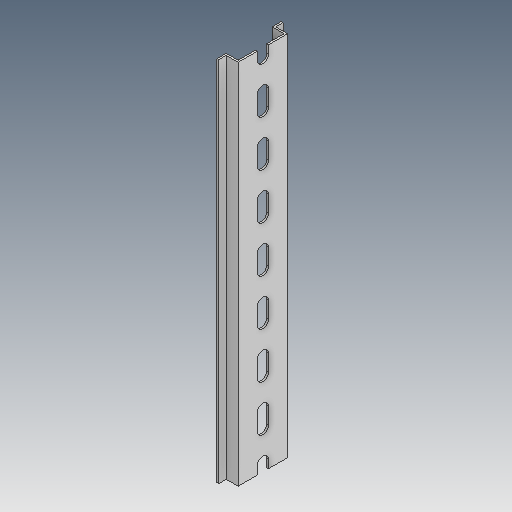
# Autodesk Inventor part: din_rail
Saved by Autodesk Inventor 2025.4 (Build 294407020, 407B)
## iProperties
Created: 2026-09-16
Part Number: din_rail
Material: Generic
Document SubType Name: Modeling
Designer: Aiden
Density: 1 g/cm^3
Appearance: Default
Author: Aiden
Autodesk Inventor part; units mm, degrees
ref_plane "YZ Plane" through (0, 0, 0) normal (1, 0, 0) x (0, 1, 0)
ref_plane "XZ Plane" through (0, 0, 0) normal (0, 1, 0) x (-1, 0, 0)
ref_plane "XY Plane" through (0, 0, 0) normal (0, 0, 1) x (1, 0, 0)
sketch "Sketch1" plane through (0, 0, 0) normal (0, 1, 0) x (-1, 0, 0)
  line L0 (0, 0) -> (0, -13.5)
  line L1 (0, -13.5) -> (6.5, -13.5)
  line L2 (6.5, -13.5) -> (6.5, -17.5)
  line L3 (1, 0) -> (1, -12.5)
  line L4 (1, -12.5) -> (7.5, -12.5)
  line L5 (7.5, -12.5) -> (7.5, -17.5)
  line L6 (7.5, -17.5) -> (6.5, -17.5)
  line L7 (1, 0) -> (0, 0) construction
  line L8 (0, 0) -> (0, 13.5)
  line L9 (0, 13.5) -> (6.5, 13.5)
  line L10 (6.5, 13.5) -> (6.5, 17.5)
  line L11 (1, 0) -> (1, 12.5)
  line L12 (1, 12.5) -> (7.5, 12.5)
  line L13 (7.5, 12.5) -> (7.5, 17.5)
  line L14 (7.5, 17.5) -> (6.5, 17.5)
  dimension "d0" = 13.5
  dimension "d1" = 1
  dimension "d2" = 7.5
  dimension "d3" = 17.5
  constraints: 30 end point, 6 symmetric about line, 3 horizontal, 2 vertical, 2 other
  measures "d0" distance of L0.start L0.end
  measures "d1" distance between parallel lines of L0 L3
  measures "d2" distance between parallel lines of L0 L5
  measures "d3" vertical distance of L2.end L0.start
extrude "Extrusion1" add sketch "Sketch1" along normal blind 200
sketch "Sketch2" plane through (-1, 0, -12.5) normal (-1, 0, 0) x (0, 0, 1)
  line L0 (0, 0) -> (25, 0) projected
  line L1 (25, 0) -> (25, 200) projected
  line L2 (0, 200) -> (25, 200) projected
  line L3 (0, 0) -> (0, 200) projected
  line L4 (25, 0) -> (25, 200) projected
  line L5 (12.5, 104.4) -> (12.5, 95.6) construction
  line L6 (30, 0) -> (30, 200) projected
  line L7 (9.4, 104.4) -> (9.4, 95.6)
  line L8 (15.6, 95.6) -> (15.6, 104.4)
  arc A0 (15.6, 104.4) -> (9.4, 104.4) centre (12.5, 104.4) ccw
  arc A1 (9.4, 95.6) -> (15.6, 95.6) centre (12.5, 95.6) ccw
  line L9 (12.5, 129.4) -> (12.5, 120.6) construction
  line L10 (9.4, 129.4) -> (9.4, 120.6)
  line L11 (15.6, 120.6) -> (15.6, 129.4)
  arc A2 (15.6, 129.4) -> (9.4, 129.4) centre (12.5, 129.4) ccw
  arc A3 (9.4, 120.6) -> (15.6, 120.6) centre (12.5, 120.6) ccw
  line L12 (12.5, 79.4) -> (12.5, 70.6) construction
  line L13 (9.4, 79.4) -> (9.4, 70.6)
  line L14 (15.6, 70.6) -> (15.6, 79.4)
  arc A4 (15.6, 79.4) -> (9.4, 79.4) centre (12.5, 79.4) ccw
  arc A5 (9.4, 70.6) -> (15.6, 70.6) centre (12.5, 70.6) ccw
  line L15 (12.5, 154.4) -> (12.5, 145.6) construction
  line L16 (9.4, 154.4) -> (9.4, 145.6)
  line L17 (15.6, 145.6) -> (15.6, 154.4)
  arc A6 (15.6, 154.4) -> (9.4, 154.4) centre (12.5, 154.4) ccw
  arc A7 (9.4, 145.6) -> (15.6, 145.6) centre (12.5, 145.6) ccw
  line L18 (12.5, 54.4) -> (12.5, 45.6) construction
  line L19 (9.4, 54.4) -> (9.4, 45.6)
  line L20 (15.6, 45.6) -> (15.6, 54.4)
  arc A8 (15.6, 54.4) -> (9.4, 54.4) centre (12.5, 54.4) ccw
  arc A9 (9.4, 45.6) -> (15.6, 45.6) centre (12.5, 45.6) ccw
  line L21 (12.5, 179.4) -> (12.5, 170.6) construction
  line L22 (9.4, 179.4) -> (9.4, 170.6)
  line L23 (15.6, 170.6) -> (15.6, 179.4)
  arc A10 (15.6, 179.4) -> (9.4, 179.4) centre (12.5, 179.4) ccw
  arc A11 (9.4, 170.6) -> (15.6, 170.6) centre (12.5, 170.6) ccw
  line L24 (12.5, 29.4) -> (12.5, 20.6) construction
  line L25 (9.4, 29.4) -> (9.4, 20.6)
  line L26 (15.6, 20.6) -> (15.6, 29.4)
  arc A12 (15.6, 29.4) -> (9.4, 29.4) centre (12.5, 29.4) ccw
  arc A13 (9.4, 20.6) -> (15.6, 20.6) centre (12.5, 20.6) ccw
  line L27 (12.5, 204.4) -> (12.5, 195.6) construction
  line L28 (9.4, 204.4) -> (9.4, 195.6)
  line L29 (15.6, 195.6) -> (15.6, 204.4)
  arc A14 (15.6, 204.4) -> (9.4, 204.4) centre (12.5, 204.4) ccw
  arc A15 (9.4, 195.6) -> (15.6, 195.6) centre (12.5, 195.6) ccw
  line L30 (12.5, 4.4) -> (12.5, -4.4) construction
  line L31 (9.4, 4.4) -> (9.4, -4.4)
  line L32 (15.6, -4.4) -> (15.6, 4.4)
  arc A16 (15.6, 4.4) -> (9.4, 4.4) centre (12.5, 4.4) ccw
  arc A17 (9.4, -4.4) -> (15.6, -4.4) centre (12.5, -4.4) ccw
  point P0 (12.5, 0)
  point P1 (12.5, 100)
  point P2 (12.5, 200)
  point P3 (25, 100)
  point P4 (12.5, 107.5)
  point P5 (12.5, 92.5)
  point P6 (12.5, 132.5)
  point P7 (12.5, 117.5)
  point P8 (12.5, 125)
  point P9 (12.5, 82.5)
  point P10 (12.5, 67.5)
  point P11 (12.5, 75)
  point P12 (12.5, 157.5)
  point P13 (12.5, 142.5)
  point P14 (12.5, 150)
  point P15 (12.5, 57.5)
  point P16 (12.5, 42.5)
  point P17 (12.5, 50)
  point P18 (12.5, 182.5)
  point P19 (12.5, 167.5)
  point P20 (12.5, 175)
  point P21 (12.5, 32.5)
  point P22 (12.5, 17.5)
  point P23 (12.5, 25)
  point P24 (12.5, 207.5)
  point P25 (12.5, 192.5)
  point P26 (12.5, 200)
  point P27 (12.5, 7.5)
  point P28 (12.5, -7.5)
  point P29 (12.5, 0)
  point P30 (9.4, 0)
  point P31 (15.6, 0)
  dimension "d6" = 6.2
  dimension "d7" = 15
  dimension "d10" = 25
  constraints: 72 end point, 38 point on circle, 18 centre point, 4 tangent, 3 midpoint, 2 parallel, 1 horizontal alignment, 1 vertical, 1 vertical alignment, 112 other
  measures "d6" distance between parallel lines of L7 L8
  measures "d7" distance of point (12.5, 107.5) point (12.5, 92.5)
  measures "d10" distance of L7.start L10.start
extrude "Extrusion2" cut sketch "Sketch2" against normal blind 15 contours L31 A16 L32 L0 | L28 A14 L29 L2 | L2 L29 A15 L28 | A0 L8 A1 L7 | A2 L11 A3 L10 | A4 L14 A5 L13 | A6 L17 A7 L16 | A8 L20 A9 L19 | A10 L23 A11 L22 | A12 L26 A13 L25
equation "\"d15\" = d7"
body "Solid1"
